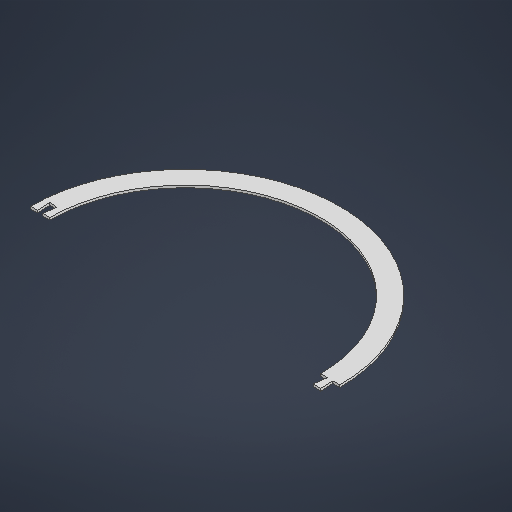
# Autodesk Inventor part: base
Saved by Autodesk Inventor 2026.2 (Build 302298000, 298)
## iProperties
Created: 2026-02-13
Part Number: base
Material: Genérico
Document SubType Name: Chapa de metal
Designer: Ian
Density: 1 g/cm^3
Appearance: Padrão
Sheet Metal Rule: Padrão
Author: Ian
Autodesk Inventor part; units mm, degrees
ref_plane "YZ Plane" through (0, 0, 0) normal (1, 0, 0) x (0, 1, 0)
ref_plane "XZ Plane" through (0, 0, 0) normal (0, 1, 0) x (-1, 0, 0)
ref_plane "XY Plane" through (0, 0, 0) normal (0, 0, 1) x (1, 0, 0)
sketch "Esboço1" plane through (0, 0, 0) normal (0, 1, 0) x (-1, 0, 0)
  arc A0 (-350, 0) -> (-247.4874, -247.4874) centre (0, 0) ccw
  arc A1 (-400, 0) -> (-282.8427, -282.8427) centre (0, 0) ccw
  circle A2 centre (0, 0) radius 400
  circle A3 centre (0, 0) radius 350
  line L0 (0, 0) -> (576.9105, 0)
  line L1 (0, 0) -> (-1224.3013, 0) construction
  line L2 (-350, 0) -> (-400, 0)
  point P0 (-282.8427, -282.8427)
  point P1 (-247.4874, -247.4874)
  point P2 (-282.8427, -282.8427)
  point P3 (400, 0)
  point P4 (350, 0)
  point P5 (-247.4874, -247.4874)
  dimension "d27" = 700
  dimension "d28" = 800
  dimension "d87" = 180
  constraints: 6 end point, 6 point on circle, 4 coincident, 3 centre point, 1 horizontal, 4 other
  measures "d27" diameter of A0
  measures "d28" diameter of A1
  measures "d87" angle of L1 L0
extrude "Extrusão1" add sketch "Esboço1" along normal blind 6 contours A0 A3 L0 A2 A1 L2
sketch "Esboço5" plane through (0, 6, 0) normal (0, 1, 0) x (1, 0, 0)
  arc A0 (400, 0) -> (-400, 0) centre (0, 0) ccw projected
  line L0 (-400, 0) -> (-350, 0) projected
  line L1 (0, 0) -> (-469.4096, 41.068)
  circle A1 centre (0, 0) radius 400
  arc A2 (350, 0) -> (-350, 0) centre (0, 0) ccw projected
  circle A3 centre (0, 0) radius 350
  line L2 (-400, 0) -> (-382, 0)
  line L3 (-382, 0) -> (-368, 0)
  line L4 (-398.4779, 34.8623) -> (-383.535, 33.555)
  line L5 (-383.535, 33.555) -> (-363.6111, 31.8118)
  line L6 (-382, 0) -> (-383.535, 33.555)
  line L7 (-368, 0) -> (-363.6111, 31.8118)
  point P0 (-348.6681, 30.5045)
  point P1 (-398.4779, 34.8623)
  point P2 (-348.6681, 30.5045)
  point P3 (-400, 0)
  dimension "d98" = -5
  dimension "d99" = 18
  dimension "d100" = 14
  dimension "d101" = 15
  dimension "d102" = 20
  constraints: 14 end point, 5 point on line, 2 coincident, 2 point on circle, 1 centre point, 3 other
  measures "d98" angle of L0 L1
  measures "d99" distance of L0.start L2.end
  measures "d100" distance of L2.end L3.end
  measures "d101" distance of L4.start L4.end
  measures "d102" distance of L4.end L5.end
extrude "Extrusão5" cut sketch "Esboço5" against normal up to surface (6 mm away) contours L1 L7 L0 L6
sketch "Esboço6" plane through (0, 6, 0) normal (0, 1, 0) x (1, 0, 0)
  arc A0 (400, 0) -> (-400, 0) centre (0, 0) ccw projected
  circle A1 centre (0, 0) radius 400
  circle A2 centre (0, 0) radius 350
  line L0 (0, 0) -> (512.6153, -44.848)
  line L1 (350, 0) -> (400, 0) projected
  line L2 (350, 0) -> (368, 0)
  line L3 (368, 0) -> (382, 0)
  line L4 (382, 0) -> (400, 0)
  line L5 (348.6681, -30.5045) -> (363.6111, -31.8118)
  line L6 (363.6111, -31.8118) -> (383.535, -33.555)
  line L7 (383.535, -33.555) -> (398.4779, -34.8623)
  line L8 (368, 0) -> (363.6111, -31.8118)
  line L9 (382, 0) -> (383.535, -33.555)
  point P0 (-398.4779, 34.8623)
  dimension "d93" = 5
  dimension "d94" = 18
  dimension "d95" = 14
  dimension "d96" = 15
  dimension "d97" = 20
  constraints: 18 end point, 6 point on line, 4 point on circle, 2 centre point, 2 coincident, 1 collinear, 6 other
  measures "d93" angle of L1 L0
  measures "d94" distance of L1.start L2.end
  measures "d95" distance of L2.end L3.end
  measures "d96" distance of L5.start L5.end
  measures "d97" distance of L5.end L6.end
extrude "Extrusão6" add sketch "Esboço6" against normal up to surface (6 mm away) contours L9 L0 L8 L1
